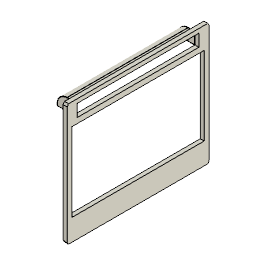
LCD mount (Autodesk Fusion 360 design; units mm, degrees)
part number: 2026-06-29-18-25-40-189
Autodesk Fusion 360 part; units mm, degrees
sketch "Sketch1" plane through (0, 0, 0) normal (1, 0, 0) x (0, 1, 0)
  line L0 (87.5, 75) -> (-87.5, 75)
  line L1 (-87.5, 75) -> (-87.5, -75)
  line L2 (-87.5, -75) -> (87.5, -75)
  line L3 (87.5, -75) -> (87.5, 75)
  line L4 (87.5, 75) -> (-87.5, -75) construction
  line L5 (-87.5, 75) -> (87.5, -75) construction
  line L6 (-87.5, 72.5134) -> (-85.8217, 75)
  line L7 (0, 75) -> (0, -75) construction
  line L8 (-87.5, 0) -> (87.5, 0) construction
  line L9 (87.5, 72.5134) -> (85.8217, 75)
  line L10 (87.5, -72.5134) -> (85.8217, -75)
  line L11 (-87.5, -72.5134) -> (-85.8217, -75)
  line L12 (81.5, 48.35) -> (-81.5, 48.35)
  line L13 (-81.5, 48.35) -> (-81.5, -48.35)
  line L14 (-81.5, -48.35) -> (81.5, -48.35)
  line L15 (81.5, -48.35) -> (81.5, 48.35)
  line L16 (81.5, 48.35) -> (-81.5, -48.35) construction
  line L17 (-81.5, 48.35) -> (81.5, -48.35) construction
  line L18 (75, 55) -> (-75, 55)
  line L19 (-75, 55) -> (-75, 70)
  line L20 (-75, 70) -> (75, 70)
  line L21 (75, 70) -> (75, 55)
  line L22 (75, 55) -> (-75, 70) construction
  line L23 (-75, 55) -> (75, 70) construction
  point P0 (0, 62.5)
  dimension "d1" = 175
  dimension "d2" = 150
  dimension "d3" = 3
  dimension "d4" = 163
  dimension "d5" = 96.7
  dimension "d8" = 150
  dimension "d9" = 15
  dimension "d10" = 5
  constraint horizontal L0
  constraint perpendicular L0 L1
  constraint parallel L0 L2
  constraint parallel L1 L3
  constraint coincident L4 origin
  constraint coincident L5 origin
  constraint coincident L1 L6.start
  constraint coincident L0 L6.end
  constraint midpoint L0 L7.start
  constraint midpoint L2 L7.end
  constraint midpoint L1 L8.start
  constraint midpoint L3 L8.end
  constraint symmetric L6.start L7 L9.start
  constraint symmetric L6.end L7 L9.end
  constraint symmetric L6.start L8 L11.start
  constraint symmetric L6.end L8 L11.end
  constraint symmetric L8 L9.start L10.start
  constraint symmetric L8 L9.end L10.end
  constraint horizontal L12
  constraint perpendicular L12 L13
  constraint parallel L12 L14
  constraint parallel L13 L15
  constraint coincident L16 origin
  constraint coincident L17 origin
  constraint horizontal L18
  constraint perpendicular L18 L19
  constraint parallel L18 L20
  constraint parallel L19 L21
  constraint coincident L22 P0
  constraint coincident L23 P0
  constraint coincident L7 P0
  measures "d1" distance of L1.end L2.end
  measures "d2" distance of L0.end L1.end
  measures "d3" distance of L6.start L6.end
  measures "d4" distance of L13.end L14.end
  measures "d5" distance of L12.end L13.end
  measures "d8" distance of L19.end L20.end
  measures "d9" distance of L18.end L19.end
  measures "d10" distance of L0 L20
extrude "Extrude1" add sketch "Sketch1" along normal blind 5 contours L0 L1 L2 L3 L6 L9 L10 L11 | L18 L19 L20 L21 makes body 1
extrude "Extrude2" cut sketch "Sketch1" along normal blind 10 contours L18 L19 L20 L21 bodies 1
sketch "Sketch2" plane through (0, 0, 0) normal (-1, 0, 0) x (0, -1, 0)
  line L0 (-75, 55) -> (-75, 70)
  line L1 (-75, 70) -> (75, 70)
  line L2 (75, 70) -> (75, 55)
  line L3 (75, 55) -> (-75, 55)
  line L4 (-81.5, -48.35) -> (-81.5, 48.35)
  line L5 (-81.5, 48.35) -> (81.5, 48.35)
  line L6 (81.5, 48.35) -> (81.5, -48.35)
  line L7 (81.5, -48.35) -> (-81.5, -48.35)
  line L8 (87.5, -72.5134) -> (87.5, 72.5134)
  line L9 (87.5, 72.5134) -> (85.8217, 75)
  line L10 (85.8217, 75) -> (-85.8217, 75)
  line L11 (-85.8217, 75) -> (-87.5, 72.5134)
  line L12 (-87.5, 72.5134) -> (-87.5, -72.5134)
  line L13 (-87.5, -72.5134) -> (-85.8217, -75)
  line L14 (-85.8217, -75) -> (85.8217, -75)
  line L15 (85.8217, -75) -> (87.5, -72.5134)
ref_plane "WorkPlane1" through (0, 75, 0) normal (0, 1, 0) x (0, 0, 1)
sketch "Sketch3" plane through (0, 75, 0) normal (0, 1, 0) x (1, 0, 0)
  line L0 (0, -55) -> (-20, -55)
  line L1 (0, -70) -> (-7.75, -70)
  spline S0 degree 1 poles (-20, -55) (-20, -57.75) knots 0 0 0.183333 0.183333
  arc A0 (-20, -57.75) -> (-7.75, -70) centre (-7.75, -57.75) ccw
  line L2 (-20, -55) -> (-20, -57.75) construction
  line L3 (0, -70) -> (0, -55)
  line L4 (0, -69.5) -> (-7.75, -69.5)
  arc A1 (-19.5, -57.75) -> (-7.75, -69.5) centre (-7.75, -57.75) ccw
  spline S1 degree 1 poles (-19.5, -55) (-19.5, -57.75) knots 0 0 0.275 0.275
  point P0 (0, -70)
  point P1 (0, -55)
  dimension "d14" = 20
  dimension "d15" = 12.25
  dimension "d16" = -0.5
  dimension "d17" = -0.5
  constraint horizontal L0
  constraint coincident P0 L1.start
  constraint horizontal L1
  constraint tangent S0 A0
  constraint tangent L1 A0
  constraint perpendicular L0 L3
  measures "d14" distance of L0.start L0.end
  measures "d15" radius of A0
extrude "Extrude3" add sketch "Sketch3" against normal blind 150 separate body contours L0 L1 S0 A0 L3 L4 A1 S1 makes body 2
extrude "Extrude4" add sketch "Sketch3" against normal blind 0.5 separate body contours L0 L3 L4 A1 S1 makes body 3
mirror "Mirror1" about plane through (0, 0, 0) normal (0, 1, 0) of bodies 3 makes body 4
fillet "Fillet1" radius 0.5 3 edges at (-3.875, 75, 70) (-16.4121, 75, 66.4121) (-20, 75, 56.375) on bodies 2
fillet "Fillet2" radius 0.1 1 edges at (-9.75, 75, 55) on bodies 3
fillet "Fillet3" radius 0.1 2 edges at (-19.8536, 74.8536, 55) (-20, -0.25, 55) on bodies 2
fillet "Fillet4" radius 0.1 1 edges at (-9.75, -75, 55) on bodies 4
fillet "Fillet5" radius 0.1 5 edges at (-3.875, -75, 70) (-16.4121, -75, 66.4121) (-20, -75, 56.425) (-19.9707, -75, 55.0293) (-19.7, -75, 55) on bodies 2
